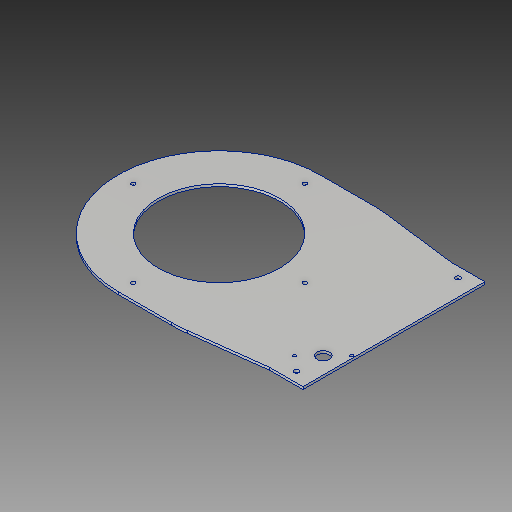
# Autodesk Inventor part: BAG motor top plate
Saved by Autodesk Inventor 2017 (Build 210142000, 142)
## iProperties
Created: 2016-10-01
Part Number: BAG motor top plate
Material: Aluminum 6061
Document SubType Name: Modeling
Designer: 15102898
Density: 2.7 g/cm^3
Appearance: Aluminum - Flat
Mass: 516.017 g
Surface Area: 1258.74 cm^2
Volume: 191.118 cm^3
Author: 15102898
Autodesk Inventor part; units mm, degrees
ref_plane "YZ Plane" through (0, 0, 0) normal (1, 0, 0) x (0, 1, 0)
ref_plane "XZ Plane" through (0, 0, 0) normal (0, 1, 0) x (-1, 0, 0)
ref_plane "XY Plane" through (0, 0, 0) normal (0, 0, 1) x (1, 0, 0)
sketch "Sketch1" plane through (0, 0, 0) normal (0, 1, 0) x (-1, 0, 0)
  line L0 (0, 0) -> (-42.0116, 0)
  line L1 (-42.0116, 0) -> (-42.0116, -228.6)
  line L2 (-42.0116, -228.6) -> (0, -228.6)
  line L3 (0, -228.6) -> (0, 0)
  circle A0 centre (-21.0058, -12.7) radius 3.175
  circle A1 centre (-21.0058, -215.9) radius 3.175
  circle A2 centre (-3.048, -28.448) radius 2.0193
  circle A3 centre (-38.9636, -64.3636) radius 2.0193
  line L4 (0, 0) -> (101.6, 12.7)
  line L5 (101.6, 12.7) -> (177.8, 12.7)
  line L6 (304.8, -114.3) -> (304.8, -114.3)
  line L7 (177.8, -241.3) -> (101.6, -241.3)
  line L8 (101.6, -241.3) -> (0, -228.6)
  circle A4 centre (177.8, -114.3) radius 76.2
  arc A5 (304.8, -114.3) -> (177.8, 12.7) centre (177.8, -114.3) ccw
  arc A6 (177.8, -241.3) -> (304.8, -114.3) centre (177.8, -114.3) ccw
  point P0 (304.8, 12.7)
  point P1 (304.8, -241.3)
  dimension "d0" = 42.0116
  dimension "d1" = 228.6
  dimension "d2" = 12.7
  dimension "d3" = 12.7
  dimension "d4" = 6.35
  dimension "d5" = 21.0058
  dimension "d6" = 21.0058
  dimension "d7" = 6.35
  dimension "d8" = 28.448
  dimension "d9" = 3.048
  dimension "d10" = 4.0386
  dimension "d11" = 4.0386
  dimension "d12" = 64.3636
  dimension "d13" = 3.048
  dimension "d21" = 152.4
  dimension "d22" = 254
  dimension "d23" = 203.2
  dimension "d24" = 101.6
  dimension "d25" = 127
  dimension "d26" = 127
  dimension "d27" = 127
  dimension "d28" = 127
  constraints: 18 end point, 7 centre point, 4 point on circle, 4 point on line, 4 tangent, 3 parallel, 2 equal length, 2 perpendicular, 1 horizontal, 1 vertical
  measures "d0" distance of L2.end L1.end
  measures "d1" distance of L1.end L0.end
  measures "d2" distance from line of L0 A0.centre
  measures "d3" distance from line of L2 A1.centre
  measures "d4" diameter of A1
  measures "d5" distance from line of L1 A0.centre
  measures "d6" distance from line of L3 A1.centre
  measures "d7" diameter of A0
  measures "d8" distance from line of L0 A2.centre
  measures "d9" distance from line of L3 A2.centre
  measures "d10" diameter of A2
  measures "d11" diameter of A3
  measures "d12" distance from line of L0 A3.centre
  measures "d13" distance from line of L1 A3.centre
  measures "d21" diameter of A4
  measures "d22" distance of point (304.8, 12.7) point (304.8, -241.3)
  measures "d23" distance of L4.end point (304.8, 12.7)
  measures "d24" distance from line of L3 L4.end
  measures "d25" radius of A5
  measures "d26" radius of A6
  measures "d27" distance from line of L5 A4.centre
  measures "d28" distance from line of L6 A4.centre
extrude "Extrusion1" add sketch "Sketch1" along normal blind 3.175
sketch "Sketch2" plane through (0, 3.175, 0) normal (0, 1, 0) x (1, 0, 0)
  circle A0 centre (21.0058, 46.4058) radius 7.9375
  line L0 (0, 228.6) -> (0, 0) projected
  line L1 (0, 0) -> (42.0116, 0) projected
  line L2 (42.0116, 228.6) -> (0, 228.6) projected
  line L3 (0, 0) -> (0, 228.6)
  line L4 (42.0116, 0) -> (42.0116, 228.6) projected
  dimension "d16" = 15.875
  dimension "d18" = 46.4058
  dimension "d31" = 21.0058
  constraints: 2 end point, 1 centre point, 1 vertical
  measures "d16" diameter of A0
  measures "d18" distance from line of L1 A0.centre
  measures "d31" distance from line of L4 A0.centre
extrude "Extrusion2" cut sketch "Sketch2" against normal blind 7.9375 contours A0
fillet "Fillet1" radius 152.4 2 edges at (-101.6, 1.5875, 12.7) (-101.6, 1.5875, -241.3)
sketch "Sketch3" plane through (0, 3.175, 0) normal (0, 1, 0) x (1, 0, 0)
  circle A0 centre (-177.8, 114.3) radius 107.95 construction
  circle A1 centre (-177.8, 114.3) radius 76.2 projected
  circle A2 centre (-177.8, 6.35) radius 2.5781
  circle A3 centre (-69.85, 114.3) radius 2.5781
  circle A4 centre (-177.8, 222.25) radius 2.5781
  circle A5 centre (-285.75, 114.3) radius 2.5781
  line L0 (-177.8, 114.3) -> (-177.8, 6.35) construction
  line L1 (-177.8, 114.3) -> (-69.85, 114.3) construction
  line L2 (-177.8, 114.3) -> (-177.8, 222.25) construction
  line L3 (-177.8, 114.3) -> (-285.75, 114.3) construction
  point P0 (0, 0)
  dimension "d33" = 215.9
  dimension "d35" = 90
  dimension "d43" = 90
  dimension "d44" = 90
  constraints: 8 end point, 5 centre point, 4 point on circle, 3 equal radius, 1 concentric, 1 vertical
  measures "d33" diameter of A0
  measures "d35" angle of L1 L0
  measures "d43" angle of L1 L2
  measures "d44" angle of L3 L2
extrude "Extrusion3" cut sketch "Sketch3" against normal blind 25.4 contours A2 | A3 | A4 | A5
body "Solid1"
